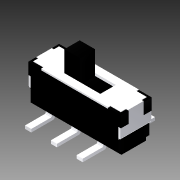
# Autodesk Inventor part: PZ_Switch_SMD
Saved by Autodesk Inventor 2015 (Build 190159000, 159)
## iProperties
Created: 2015-11-10
Part Number: PZ_Switch_SMD
Material: Genérico
Document SubType Name: Modeling
Designer: X1
Density: 1 g/cm^3
Appearance: Valor por defecto
Mass: 0.100609 g
Surface Area: 1.76996 cm^2
Volume: 0.100609 cm^3
Author: X1
Autodesk Inventor part; units mm, degrees
ref_plane "YZ Plane" through (0, 0, 0) normal (1, 0, 0) x (0, 1, 0)
ref_plane "XZ Plane" through (0, 0, 0) normal (0, 1, 0) x (-1, 0, 0)
ref_plane "XY Plane" through (0, 0, 0) normal (0, 0, 1) x (1, 0, 0)
sketch "Boceto1" plane through (0, 0, 0) normal (0, 0, 1) x (1, 0, 0)
  line L0 (-5.95, 0) -> (5.95, 0) projected
  line L1 (0, -2.1) -> (0, 2.1) projected
  line L2 (4.25, 1.5) -> (-4.25, 1.5)
  line L3 (-4.25, 1.5) -> (-4.25, -1.5)
  line L4 (-4.25, -1.5) -> (4.25, -1.5)
  line L5 (4.25, -1.5) -> (4.25, 1.5)
  point P0 (0, 0)
  dimension "d0" = 8.5
  dimension "d1" = 3
  constraints: 8 end point, 2 parallel, 1 horizontal, 1 perpendicular, 2 other
  measures "d0" distance of L4.end L3.end
  measures "d1" distance of L3.end L2.end
extrude "Extrusión1" add sketch "Boceto1" along normal blind 3.5
sketch "Boceto2" plane through (-4.25, -1.5, 0) normal (0, -1, 0) x (1, 0, 0)
  line L0 (0, 0) -> (8.5, 0) projected
  line L1 (8.5, 0) -> (8.5, 3.5) projected
  line L2 (0, 3.5) -> (8.5, 3.5) projected
  line L3 (0, 0) -> (0, 3.5) projected
  line L4 (0, 3.5) -> (-0.25, 3.5)
  line L5 (-0.25, 3.5) -> (-0.25, 2.5)
  line L6 (-0.25, 2.5) -> (0, 2.5)
  line L7 (8.5, 3.5) -> (8.75, 3.5)
  line L8 (8.75, 3.5) -> (8.75, 2.5)
  line L9 (8.75, 2.5) -> (8.5, 2.5)
  line L10 (1.5, 3.5) -> (1.5, 3.3)
  line L11 (1.5, 3.3) -> (7, 3.3)
  line L12 (7, 3.3) -> (7, 3.5)
  point P0 (4.25, 0)
  dimension "d4" = 0.25
  dimension "d5" = 1
  dimension "d6" = 0.25
  dimension "d7" = 0.2
  dimension "d8" = 1.5
  dimension "d9" = 1.5
  constraints: 18 end point, 6 perpendicular, 4 point on line, 3 horizontal
  measures "d4" distance of L2.start L4.end
  measures "d5" distance of L4.end L5.end
  measures "d6" distance of L1.end L7.end
  measures "d7" distance of L10.start L10.end
  measures "d8" distance between parallel lines of L10 L3
  measures "d9" distance between parallel lines of L1 L12
extrude "Extrusión2" add sketch "Boceto2" against normal blind 0.75 contours L6 L5 L4 L3 | L1 L7 L8 L9
mirror "Simetría1" about plane through (0, 0, 0) normal (0, 1, 0) of "Extrusión2"
sketch "Boceto3" plane through (0, 0, 3.5) normal (0, 0, 1) x (1, 0, 0)
  line L0 (4.5, 1.5) -> (-4.5, 1.5) projected
  line L1 (-4.5, 1.5) -> (-4.5, 0.75) projected
  line L2 (-4.5, 0.75) -> (-4.25, 0.75) projected
  line L3 (-4.25, 0.75) -> (-4.25, -0.75) projected
  line L4 (-4.5, -0.75) -> (-4.25, -0.75) projected
  line L5 (-4.5, -1.5) -> (-4.5, -0.75) projected
  line L6 (4.5, -1.5) -> (-4.5, -1.5) projected
  line L7 (4.5, -1.5) -> (4.5, -0.75) projected
  line L8 (4.25, -0.75) -> (4.5, -0.75) projected
  line L9 (4.25, -0.75) -> (4.25, 0.75) projected
  line L10 (4.25, 0.75) -> (4.5, 0.75) projected
  line L11 (4.5, 1.5) -> (4.5, 0.75) projected
  line L12 (-4.25, 0.75) -> (-4.25, 1.25)
  line L13 (-4.25, 1.25) -> (-3.25, 1.25)
  line L14 (-3.25, 1.25) -> (-3.25, 1.5)
  line L15 (4.25, 1.5) -> (-4.25, 1.5) projected
  line L16 (-4.25, -0.75) -> (-4.25, -1.25)
  line L17 (-4.25, -1.25) -> (-3.25, -1.25)
  line L18 (-3.25, -1.25) -> (-3.25, -1.5)
  line L19 (0, -2.1) -> (0, 2.1) projected
  line L20 (4.25, 0.75) -> (4.25, 1.25)
  line L21 (4.25, 1.25) -> (3.25, 1.25)
  line L22 (3.25, 1.25) -> (3.25, 1.5)
  line L23 (4.25, -0.75) -> (4.25, -1.25)
  line L24 (4.25, -1.25) -> (3.25, -1.25)
  line L25 (3.25, -1.25) -> (3.25, -1.5)
  point P0 (0, 0)
  dimension "d12" = 0.25
  dimension "d13" = 1
  dimension "d14" = 0.5
  dimension "d15" = 0.5
  dimension "d17" = 1
  dimension "d18" = 0.25
  dimension "d19" = 0.5
  dimension "d20" = 1
  dimension "d21" = 0.25
  dimension "d22" = 0.5
  dimension "d23" = 1
  dimension "d24" = 0.25
  constraints: 24 end point, 5 perpendicular, 4 point on line, 3 horizontal
  measures "d12" distance from line of L0 L12.end
  measures "d13" distance of L12.end L13.end
  measures "d14" distance of L2.end L12.end
  measures "d15" distance of L3.end L16.end
  measures "d17" distance of L16.end L17.end
  measures "d18" distance of L17.end L18.end
  measures "d19" distance of L9.end L20.end
  measures "d20" distance of L20.end L21.end
  measures "d21" distance of L21.end L22.end
  measures "d22" distance of L8.start L23.end
  measures "d23" distance of L23.end L24.end
  measures "d24" distance of L24.end L25.end
extrude "Extrusión3" add sketch "Boceto3" along normal blind 0.1 contours L11 L10 L20 L21 L22 L0 | L8 L7 L6 L25 L24 L23 | L14 L13 L12 L2 L1 L0 | L6 L5 L4 L16 L17 L18
sketch "Boceto4" plane through (-4.25, -1.5, 0) normal (-1, 0, 0) x (0, 0, 1)
  line L0 (3.5, 2.25) -> (2.5, 2.25) projected
  line L1 (2.5, 2.25) -> (2.5, 3) projected
  line L2 (0, 3) -> (2.5, 3) projected
  line L3 (0, 3) -> (0, 0) projected
  line L4 (0, 0) -> (2.5, 0) projected
  line L5 (2.5, 0) -> (2.5, 0.75) projected
  line L6 (2.5, 0.75) -> (3.5, 0.75) projected
  line L7 (3.5, 2.25) -> (3.5, 0.75) projected
  line L8 (1.5, 3) -> (1.5, 0)
  line L9 (2.5, 3) -> (2.5, 2.25) projected
  line L10 (2.5, 2.99) -> (1.5, 2.99)
  line L11 (2.5, 0.01) -> (1.5, 0.01)
  point P0 (0, 1.5)
  dimension "d27" = 1
  dimension "d40" = 0.01
  dimension "d41" = 0.01
  constraints: 6 end point, 6 point on line, 3 perpendicular
  measures "d27" distance between parallel lines of L1 L8
  measures "d40" distance between parallel lines of L2 L10
  measures "d41" distance between parallel lines of L4 L11
extrude "Extrusión4" add sketch "Boceto4" along normal blind 0.2 contours L7 L6 L5 L11 L8 L10 L1 L0 | L10 L8 L2 L1 | L5 L4 L8 L11
mirror "Simetría2" about plane through (0, 0, 0) normal (1, 0, 0) of "Extrusión4"
sketch "Boceto6" plane through (0, 0, 3.5) normal (0, 0, 1) x (1, 0, 0)
  line L0 (-3.25, -1.25) -> (-3.25, -1.5) projected
  line L1 (3.25, -1.5) -> (-3.25, -1.5) projected
  line L2 (3.25, -1.5) -> (3.25, -1.25) projected
  line L3 (3.25, -1.25) -> (4.25, -1.25) projected
  line L4 (4.25, -1.25) -> (4.25, -0.75) projected
  line L5 (4.45, -0.75) -> (4.25, -0.75) projected
  line L6 (4.45, -0.75) -> (4.45, 0.75) projected
  line L7 (4.25, 0.75) -> (4.45, 0.75) projected
  line L8 (4.25, 0.75) -> (4.25, 1.25) projected
  line L9 (4.25, 1.25) -> (3.25, 1.25) projected
  line L10 (3.25, 1.25) -> (3.25, 1.5) projected
  line L11 (3.25, 1.5) -> (-3.25, 1.5) projected
  line L12 (-3.25, 1.5) -> (-3.25, 1.25) projected
  line L13 (-3.25, 1.25) -> (-4.25, 1.25) projected
  line L14 (-4.25, 1.25) -> (-4.25, 0.75) projected
  line L15 (-4.45, 0.75) -> (-4.25, 0.75) projected
  line L16 (-4.45, -0.75) -> (-4.45, 0.75) projected
  line L17 (-4.25, -0.75) -> (-4.45, -0.75) projected
  line L18 (-4.25, -0.75) -> (-4.25, -1.25) projected
  line L19 (-4.25, -1.25) -> (-3.25, -1.25) projected
  line L20 (-3.25, 1.49) -> (3.25, 1.49)
  line L21 (-3.25, -1.49) -> (3.25, -1.49)
  point P0 (0, 0)
  dimension "d30" = 0.01
  dimension "d31" = 0.01
  constraints: 4 end point, 4 point on line, 1 parallel, 1 perpendicular
  measures "d30" distance between parallel lines of L11 L20
  measures "d31" distance between parallel lines of L21 L1
extrude "Extrusión5" add sketch "Boceto6" along normal blind 0.15 contours L19 L18 L17 L16 L15 L14 L13 L12 L20 L10 L9 L8 L7 L6 L5 L4 L3 L2 L21 L0
fillet "Empalme1" radius 0.1 2 edges at (4.45, 0, 1.5) (4.25, 0, 1.5)
fillet "Empalme2" radius 0.1 2 edges at (-4.45, 0, 1.5) (-4.25, 0, 1.5)
sketch "Boceto7" plane through (0, 0, 3.65) normal (0, 0, 1) x (1, 0, 0)
  line L0 (-6.3, 0) -> (6.3, 0) projected
  line L1 (0, -2.1) -> (0, 2.1) projected
  line L2 (-1.75, 0.75) -> (1.75, 0.75)
  line L3 (1.75, 0.75) -> (1.75, -0.75)
  line L4 (1.75, -0.75) -> (-1.75, -0.75)
  line L5 (-1.75, -0.75) -> (-1.75, 0.75)
  point P0 (0, 0)
  dimension "d36" = 3.5
  dimension "d37" = 1.5
  constraints: 8 end point, 2 parallel, 1 horizontal, 1 perpendicular, 2 other
  measures "d36" distance of L3.end L4.end
  measures "d37" distance of L2.end L3.end
extrude "Extrusión6" cut sketch "Boceto7" against normal blind 0.25
extrude "Extrusión7" cut sketch "Boceto4" along normal blind 0.25 contours L10 L8 L2 L1 | L5 L4 L8 L11
mirror "Simetría3" about plane through (0, 0, 0) normal (1, 0, 0) of "Extrusión7"
sketch "Boceto8" plane through (0, 0, 3.4) normal (0, 0, 1) x (1, 0, 0)
  line L0 (-1.75, 0.75) -> (1.75, 0.75) projected
  line L1 (-1.75, -0.75) -> (-1.75, 0.75) projected
  line L2 (1.75, -0.75) -> (-1.75, -0.75) projected
  line L3 (1.75, 0.75) -> (1.75, -0.75) projected
  line L4 (-0.25, 0.75) -> (-0.25, -0.75)
  point P0 (0, 0)
  dimension "d44" = 1.5
  constraints: 2 end point, 2 point on line, 1 perpendicular
  measures "d44" distance between parallel lines of L4 L1
extrude "Extrusión8" add sketch "Boceto8" along normal blind 2.25 contours L0 L4 L2 L1
sketch "Boceto9" plane through (0, 0, 0) normal (0, 0, -1) x (-1, 0, 0)
  line L0 (-4.25, 1.5) -> (4.25, 1.5) projected
  line L1 (-4.25, -1.5) -> (-4.25, 1.5) projected
  line L2 (4.25, -1.5) -> (-4.25, -1.5) projected
  line L3 (4.25, 1.5) -> (4.25, -1.5) projected
  line L4 (4.25, -1.2) -> (-4.25, -1.2)
  line L5 (4.25, 1.2) -> (-4.25, 1.2)
  point P0 (0, 0)
  dimension "d47" = 0.3
  dimension "d48" = 0.3
  constraints: 4 end point, 4 point on line, 2 perpendicular
  measures "d47" distance between parallel lines of L2 L4
  measures "d48" distance between parallel lines of L0 L5
extrude "Extrusión9" cut sketch "Boceto9" against normal blind 0.3 contours L0 L3 L5 L1 | L4 L3 L2 L1
sketch "Boceto10" plane through (0, 0, 0.3) normal (0, 0, -1) x (-1, 0, 0)
  line L0 (4.25, 1.2) -> (-4.25, 1.2) projected
  line L1 (4.25, 1.2) -> (-4.25, 1.2) projected
  line L2 (-4.25, -1.2) -> (-4.25, 1.2) projected
  line L3 (-4.25, -1.2) -> (4.25, -1.2) projected
  line L4 (4.25, 1.2) -> (4.25, -1.2) projected
  line L5 (6.3, 0) -> (-6.3, 0) projected
  line L6 (0, -2.1) -> (0, 2.1) projected
  line L7 (-3.25, 1.5) -> (3.25, 1.5) projected
  line L8 (0.3, 1.5) -> (-0.3, 1.5)
  line L9 (-0.3, 1.5) -> (-0.3, 1.2)
  line L10 (0.3, 1.5) -> (0.3, 1.2)
  line L11 (2.2, 1.2) -> (2.2, 1.5)
  line L12 (2.8, 1.2) -> (2.8, 1.5)
  line L13 (2.8, 1.5) -> (2.2, 1.5)
  line L14 (-2.2, 1.5) -> (-2.2, 1.2)
  line L15 (-2.2, 1.5) -> (-2.8, 1.5)
  line L16 (-2.8, 1.5) -> (-2.8, 1.2)
  point P0 (0, 0)
  dimension "d51" = 0.6
  dimension "d52" = 0.6
  dimension "d54" = 1.9
  dimension "d55" = 0.6
  dimension "d56" = 1.9
  constraints: 18 end point, 12 point on line, 6 perpendicular, 1 collinear, 1 other
  measures "d51" distance of L8.start L8.end
  measures "d52" distance between parallel lines of L11 L12
  measures "d54" distance between parallel lines of L10 L11
  measures "d55" distance of L14.start L15.end
  measures "d56" distance between parallel lines of L9 L14
extrude "Extrusión10" add sketch "Boceto10" along normal blind 0.5 contours L0 L11 L7 L12 | L0 L6 L7 L10 | L0 L9 L7 L6 | L16 L7 L14 L0
sketch "Boceto11" plane through (-3.25, 1.5, 3.5) normal (0, 1, 0) x (1, 0, 0)
  line L0 (7.5, 3.2) -> (6.05, 3.2) projected
  line L1 (6.05, 3.2) -> (6.05, 3.7) projected
  line L2 (5.45, 3.7) -> (6.05, 3.7) projected
  line L3 (5.45, 3.2) -> (5.45, 3.7) projected
  line L4 (5.45, 3.2) -> (3.55, 3.2) projected
  line L5 (3.55, 3.2) -> (3.55, 3.7) projected
  line L6 (2.95, 3.7) -> (3.55, 3.7) projected
  line L7 (2.95, 3.2) -> (2.95, 3.7) projected
  line L8 (1.05, 3.2) -> (1.05, 3.7) projected
  line L9 (0.45, 3.7) -> (1.05, 3.7) projected
  line L10 (0.45, 3.2) -> (0.45, 3.7) projected
  line L11 (0.45, 3.2) -> (-1, 3.2) projected
  line L12 (-1, 3.2) -> (-1, 2.1) projected
  arc A0 (-1.1, 2) -> (-1, 2.1) centre (-1.1, 2.1) ccw projected
  line L13 (-1.1, 2) -> (-1, 2) projected
  line L14 (-1, 2) -> (-1, 1) projected
  line L15 (-1.25, 1) -> (-1, 1) projected
  line L16 (-1.25, 1) -> (-1.25, -0.1) projected
  line L17 (0, -0.1) -> (-1.25, -0.1) projected
  line L18 (0, 0) -> (0, -0.1) projected
  line L19 (6.5, 0) -> (0, 0) projected
  line L20 (6.5, 0) -> (6.5, -0.1) projected
  line L21 (7.75, -0.1) -> (6.5, -0.1) projected
  line L22 (7.75, 1) -> (7.75, -0.1) projected
  line L23 (7.5, 1) -> (7.75, 1) projected
  line L24 (7.5, 1) -> (7.5, 2) projected
  line L25 (7.5, 2) -> (7.6, 2) projected
  arc A1 (7.5, 2.1) -> (7.6, 2) centre (7.6, 2.1) ccw projected
  line L26 (7.5, 3.2) -> (7.5, 2.1) projected
  line L27 (3.55, 3.2) -> (2.95, 3.2)
  line L28 (6.05, 3.2) -> (5.45, 3.2)
  line L29 (6.05, 3.4) -> (5.45, 3.4)
  line L30 (3.55, 3.4) -> (2.95, 3.4)
  line L31 (0.45, 3.5) -> (0.45, 3.7) projected
  line L32 (1.05, 3.5) -> (1.05, 3.7) projected
  line L33 (1.05, 3.2) -> (0.45, 3.2)
  line L34 (1.05, 3.4) -> (0.45, 3.4)
  point P0 (3.25, 3.5)
  dimension "d59" = 0.3
  dimension "d60" = 0.3
  dimension "d65" = 0.3
  constraints: 12 end point, 2 centre point, 2 perpendicular, 2 point on line, 1 horizontal
  measures "d59" distance between parallel lines of L29 L2
  measures "d60" distance between parallel lines of L30 L6
  measures "d65" distance between parallel lines of L9 L34
extrude "Extrusión11" add sketch "Boceto11" along normal blind 2 contours L29 L3 L2 L1 | L30 L7 L6 L5 | L10 L9 L8 L34
extrude "Extrusión12" add sketch "Boceto11" along normal blind 0.0001 contours L27 L7 L30 L5 | L28 L3 L29 L1 | L10 L34 L8 L33
mirror "Simetría4" about plane through (0, 0, 0) normal (0, 1, 0) of "Extrusión10", "Extrusión11", "Extrusión12"
fillet "Empalme3" radius 0.1 6 edges at (2.5, -1.5001, 0.1) (0, -1.5001, 0.1) (-2.5, -1.5001, 0.1) (2.5, 1.5001, 0.1) (0, 1.5001, 0.1) (-2.5, 1.5001, 0.1)
fillet "Empalme4" radius 0.2 6 edges at (2.5, 1.2, -0.2) (2.5, -1.2, -0.2) (0, -1.2, -0.2) (-2.5, -1.2, -0.2) (0, 1.2, -0.2) (-2.5, 1.2, -0.2)
